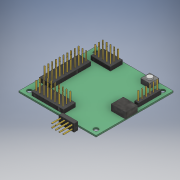
# Autodesk Inventor part: multiwii
Saved by Autodesk Inventor 2017 (Build 210142000, 142)
## iProperties
Created: 2016-12-26
Part Number: multiwii
Material: Ogólny
Document SubType Name: Modeling
Designer: Kuba01
Density: 1 g/cm^3
Appearance: Domyślna
Author: Kuba01
Autodesk Inventor part; units mm, degrees
ref_plane "YZ Plane" through (0, 0, 0) normal (1, 0, 0) x (0, 1, 0)
ref_plane "XZ Plane" through (0, 0, 0) normal (0, 1, 0) x (-1, 0, 0)
ref_plane "XY Plane" through (0, 0, 0) normal (0, 0, 1) x (1, 0, 0)
sketch "Szkic1" plane through (0, 0, 0) normal (0, 0, 1) x (1, 0, 0)
  line L0 (-25.5, 25.5) -> (25.5, 25.5)
  line L1 (25.5, 25.5) -> (25.5, -25.5)
  line L2 (25.5, -25.5) -> (-25.5, -25.5)
  line L3 (-25.5, -25.5) -> (-25.5, 25.5)
  circle A0 centre (-22, 22) radius 1.5
  circle A1 centre (-22, -22) radius 1.5
  circle A2 centre (22, -22) radius 1.5
  circle A3 centre (22, 22) radius 1.5
  point P0 (0, 0)
  point P1 (0, 25.5)
  point P2 (-25.5, 0)
  dimension "d0" = 51
  dimension "d1" = 51
  dimension "d2" = 3
  dimension "d3" = 3.5
  dimension "d4" = 3.5
  dimension "d7" = 360
  constraints: 8 end point, 4 centre point, 2 midpoint, 2 parallel, 1 horizontal, 1 horizontal alignment, 1 perpendicular, 1 vertical alignment, 9 other
  measures "d0" distance between parallel lines of L2 L0
  measures "d1" distance between parallel lines of L1 L3
  measures "d2" diameter of A0
  measures "d3" distance from line of L3 A0.centre
  measures "d4" distance from line of L0 A0.centre
extrude "Wyciągnięcie proste1" add sketch "Szkic1" along normal blind 1
sketch "Szkic2" plane through (0, 0, 1) normal (0, 0, 1) x (1, 0, 0)
  line L0 (-19.5, 24) -> (-6.5, 24)
  line L1 (-6.5, 24) -> (-6.5, 16)
  line L2 (-6.5, 16) -> (-19.5, 16)
  line L3 (-19.5, 16) -> (-19.5, 24)
  line L4 (-24, 12.5) -> (-16, 12.5)
  line L5 (-16, 12.5) -> (-16, -13.5)
  line L6 (-16, -13.5) -> (-24, -13.5)
  line L7 (-24, -13.5) -> (-24, 12.5)
  line L8 (2.5, -16) -> (2.5, -24)
  line L9 (2.5, -24) -> (-18.5, -24)
  line L10 (21, 19.5) -> (23.5, 19.5)
  line L11 (23.5, 19.5) -> (23.5, 4.5)
  line L12 (23.5, 4.5) -> (21, 4.5)
  line L13 (21, 4.5) -> (21, 19.5)
  line L14 (-25.5, 25.5) -> (-25.5, -25.5) projected
  line L15 (25.5, 25.5) -> (-25.5, 25.5) projected
  line L16 (2.5, -16) -> (-18.5, -16)
  line L17 (-18.5, -16) -> (-18.5, -24)
  line L18 (-25.5, -25.5) -> (25.5, -25.5) projected
  line L19 (25.5, -25.5) -> (25.5, 25.5) projected
  point P0 (0, 0)
  dimension "d11" = 8
  dimension "d12" = 13
  dimension "d13" = 6
  dimension "d14" = 1.5
  dimension "d15" = 26
  dimension "d16" = 8
  dimension "d17" = 13
  dimension "d18" = 1.5
  dimension "d22" = 8
  dimension "d23" = 21
  dimension "d24" = 7
  dimension "d25" = 1.5
  dimension "d26" = 15
  dimension "d27" = 2.5
  dimension "d28" = 2
  dimension "d29" = 6
  constraints: 32 end point, 6 parallel, 4 horizontal, 4 perpendicular
  measures "d11" distance between parallel lines of L2 L0
  measures "d12" distance between parallel lines of L1 L3
  measures "d13" distance between parallel lines of L14 L3
  measures "d14" distance between parallel lines of L15 L0
  measures "d15" distance between parallel lines of L6 L4
  measures "d16" distance between parallel lines of L5 L7
  measures "d17" distance between parallel lines of L15 L4
  measures "d18" distance between parallel lines of L14 L7
  measures "d22" distance between parallel lines of L9 L16
  measures "d23" distance between parallel lines of L8 L17
  measures "d24" distance between parallel lines of L14 L17
  measures "d25" distance between parallel lines of L18 L9
  measures "d26" distance between parallel lines of L12 L10
  measures "d27" distance between parallel lines of L11 L13
  measures "d28" distance between parallel lines of L19 L11
  measures "d29" distance between parallel lines of L10 L15
extrude "Wyciągnięcie proste2" add sketch "Szkic2" along normal blind 2.5 contours L0 L1 L2 L3 | L4 L5 L6 L7 | L8 L9 L17 L16 | L10 L11 L12 L13
sketch "Szkic3" plane through (0, 0, 3.5) normal (0, 0, 1) x (1, 0, 0)
  line L0 (-19.5, 24) -> (-19.5, 16) projected
  line L1 (-6.5, 24) -> (-19.5, 24) projected
  line L2 (-19.5, 24) -> (-19.5, 16) projected
  line L3 (-19.5, 16) -> (-6.5, 16) projected
  line L4 (-6.5, 16) -> (-6.5, 24) projected
  line L5 (-16, 12.5) -> (-24, 12.5) projected
  line L6 (-24, 12.5) -> (-24, -13.5) projected
  line L7 (-24, -13.5) -> (-16, -13.5) projected
  line L8 (-16, -13.5) -> (-16, 12.5) projected
  line L9 (2.5, -24) -> (2.5, -16) projected
  line L10 (2.5, -16) -> (-18.5, -16) projected
  line L11 (-18.5, -16) -> (-18.5, -24) projected
  line L12 (-18.5, -24) -> (2.5, -24) projected
  line L13 (23.5, 19.5) -> (21, 19.5) projected
  line L14 (21, 19.5) -> (21, 4.5) projected
  line L15 (21, 4.5) -> (23.5, 4.5) projected
  line L16 (23.5, 4.5) -> (23.5, 19.5) projected
  line L17 (-18.5, 23) -> (-17.9998, 23)
  line L18 (-17.9998, 23) -> (-17.9998, 22.5)
  line L19 (-17.9998, 22.5) -> (-18.5, 22.5)
  line L20 (-18.5, 22.5) -> (-18.5, 23)
  line L21 (-23, 11.5) -> (-22.5, 11.5)
  line L22 (-22.5, 11.5) -> (-22.5, 11)
  line L23 (-22.5, 11) -> (-23, 11)
  line L24 (-23, 11) -> (-23, 11.5)
  line L25 (-17.5, -17) -> (-17, -17)
  line L26 (-17, -17) -> (-17, -17.5)
  line L27 (-17, -17.5) -> (-17.5, -17.5)
  line L28 (-17.5, -17.5) -> (-17.5, -17)
  line L29 (22, 18.5) -> (22.5, 18.5)
  line L30 (22.5, 18.5) -> (22.5, 18)
  line L31 (22.5, 18) -> (22, 18)
  line L32 (22, 18) -> (22, 18.5)
  point P0 (0, 0)
  dimension "d32" = 0.5
  dimension "d33" = 0.5001
  dimension "d34" = 1
  dimension "d35" = 1
  dimension "d36" = 0.5
  dimension "d37" = 0.5
  dimension "d38" = 1
  dimension "d39" = 1
  dimension "d40" = 0.5
  dimension "d41" = 0.5
  dimension "d42" = 1
  dimension "d43" = 1
  dimension "d44" = 0.5
  dimension "d45" = 0.5
  dimension "d46" = 1
  dimension "d47" = 1
  constraints: 32 end point, 8 parallel, 4 horizontal, 4 perpendicular
  measures "d32" distance between parallel lines of L19 L17
  measures "d33" distance between parallel lines of L20 L18
  measures "d34" distance between parallel lines of L1 L17
  measures "d35" distance between parallel lines of L0 L20
  measures "d36" distance between parallel lines of L22 L24
  measures "d37" distance between parallel lines of L21 L23
  measures "d38" distance between parallel lines of L5 L21
  measures "d39" distance between parallel lines of L6 L24
  measures "d40" distance of L26.end L27.end
  measures "d41" distance of L25.end L26.end
  measures "d42" distance between parallel lines of L11 L28
  measures "d43" distance between parallel lines of L10 L25
  measures "d44" distance of L30.end L31.end
  measures "d45" distance between parallel lines of L31 L29
  measures "d46" distance between parallel lines of L13 L29
  measures "d47" distance between parallel lines of L32 L14
extrude "Wyciągnięcie proste3" add sketch "Szkic3" along normal blind 6 contours L17 L18 L19 L20
pattern_linear "Szyk prostokątny1" count 3 spacing 2.5 along (0, -1, 0) count 5 spacing 2.5 along (1, 0, 0) of "Wyciągnięcie proste3"
extrude "Wyciągnięcie proste4" add sketch "Szkic3" along normal blind 6 contours L21 L22 L23 L24
pattern_linear "Szyk prostokątny2" count 3 spacing 2.5 along (1, 0, 0) count 10 spacing 2.5 along (0, -1, 0) of "Wyciągnięcie proste4"
extrude "Wyciągnięcie proste5" add sketch "Szkic3" along normal blind 6 contours L25 L26 L27 L28
pattern_linear "Szyk prostokątny3" count 3 spacing 2.5 along (0, -1, 0) count 8 spacing 2.5 along (1, 0, 0) of "Wyciągnięcie proste5"
extrude "Wyciągnięcie proste6" add sketch "Szkic3" along normal blind 6 contours L29 L30 L31 L32
pattern_linear "Szyk prostokątny4" count 6 spacing 2.5 along (0, -1, 0) of "Wyciągnięcie proste6"
sketch "Szkic4" plane through (0, 0, 1) normal (0, 0, 1) x (1, 0, 0)
  line L0 (16.5, 1.5) -> (26, 1.5)
  line L1 (26, 1.5) -> (26, -6.5)
  line L2 (26, -6.5) -> (16.5, -6.5)
  line L3 (16.5, -6.5) -> (16.5, 1.5)
  line L4 (-25.5, -25.5) -> (25.5, -25.5) projected
  line L5 (25.5, -25.5) -> (25.5, 25.5) projected
  point P0 (0, 0)
  dimension "d77" = 19
  dimension "d78" = 8
  dimension "d79" = 9
  dimension "d80" = 9.5
  constraints: 8 end point, 2 parallel, 1 horizontal, 1 perpendicular
  measures "d77" distance between parallel lines of L2 L4
  measures "d78" distance between parallel lines of L0 L2
  measures "d79" distance between parallel lines of L3 L5
  measures "d80" distance between parallel lines of L1 L3
extrude "Wyciągnięcie proste7" add sketch "Szkic4" along normal blind 4
sketch "Szkic5" plane through (0, 0, 1) normal (0, 0, 1) x (1, 0, 0)
  line L0 (10.5, 25) -> (16.5, 25)
  line L1 (16.5, 25) -> (16.5, 19)
  line L2 (16.5, 19) -> (10.5, 19)
  line L3 (10.5, 19) -> (10.5, 25)
  line L4 (25.5, 1.5) -> (25.5, 25.5) projected
  line L5 (25.5, 25.5) -> (-25.5, 25.5) projected
  point P0 (0, 0)
  dimension "d83" = 6
  dimension "d84" = 6
  dimension "d85" = 9
  dimension "d86" = 0.5
  constraints: 8 end point, 2 parallel, 1 horizontal, 1 perpendicular
  measures "d83" distance of L1.end L2.end
  measures "d84" distance of L0.end L1.end
  measures "d85" distance between parallel lines of L4 L1
  measures "d86" distance between parallel lines of L5 L0
extrude "Wyciągnięcie proste8" add sketch "Szkic5" along normal blind 3
sketch "Szkic6" plane through (0, 0, 4) normal (0, 0, 1) x (1, 0, 0)
  line L0 (10.5, 25) -> (10.5, 19) projected
  line L1 (16.5, 19) -> (16.5, 25) projected
  line L2 (16.5, 25) -> (10.5, 25) projected
  line L3 (10.5, 19) -> (16.5, 19) projected
  circle A0 centre (13.5, 22) radius 1.75
  point P0 (0, 0)
  dimension "d89" = 3.5
  constraints: 1 centre point
  measures "d89" diameter of A0
extrude "Wyciągnięcie proste9" add sketch "Szkic6" along normal blind 1 contours A0
sketch "Szkic7" plane through (-25.5, -25.5, 0) normal (0, -1, 0) x (1, 0, 0)
  line L0 (51, 0) -> (0, 0) projected
  line L1 (51, 0) -> (51, 1) projected
  line L2 (29, 3) -> (39, 3)
  line L3 (39, 3) -> (39, -2)
  line L4 (39, -2) -> (29, -2)
  line L5 (29, -2) -> (29, 3)
  point P0 (25.5, 0)
  dimension "d92" = 5
  dimension "d93" = 10
  dimension "d94" = 12
  dimension "d95" = 2
  constraints: 8 end point, 2 parallel, 1 horizontal, 1 perpendicular
  measures "d92" distance between parallel lines of L4 L2
  measures "d93" distance between parallel lines of L3 L5
  measures "d94" distance between parallel lines of L3 L1
  measures "d95" distance between parallel lines of L0 L4
extrude "Wyciągnięcie proste10" add sketch "Szkic7" along normal blind 2.5
sketch "Szkic8" plane through (-25.5, -28, 0) normal (0, -1, 0) x (1, 0, 0)
  line L0 (30, 2) -> (30.5, 2)
  line L1 (30.5, 2) -> (30.5, 1.5)
  line L2 (30.5, 1.5) -> (30, 1.5)
  line L3 (30, 1.5) -> (30, 2)
  line L4 (29, 3) -> (29, -2) projected
  line L5 (39, 3) -> (29, 3) projected
  point P0 (25.5, 0)
  dimension "d98" = 0.5
  dimension "d99" = 0.5
  dimension "d100" = 1
  dimension "d101" = 1
  constraints: 8 end point, 2 parallel, 1 horizontal, 1 perpendicular
  measures "d98" distance of L1.end L2.end
  measures "d99" distance of L0.end L1.end
  measures "d100" distance between parallel lines of L4 L3
  measures "d101" distance between parallel lines of L5 L0
extrude "Wyciągnięcie proste11" add sketch "Szkic8" along normal blind 6
pattern_linear "Szyk prostokątny5" count 4 spacing 2.5 along (1, 0, 0) count 2 spacing 2.5 along (0, 0, -1) of "Wyciągnięcie proste11"
